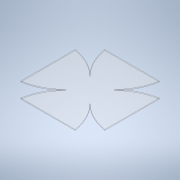
# Autodesk Inventor part: IMPRESION SIN PINES
Saved by Autodesk Inventor 2020 (Build 240168000, 168)
## iProperties
Created: 2021-11-17
Part Number: IMPRESION SIN PINES
Material: Plástico PET
Document SubType Name: Modeling
Designer: MATT
Density: 1.541 g/cm^3
Appearance: Policarbonato - Claro
Author: MATT
Autodesk Inventor part; units mm, degrees
ref_plane "YZ Plane" through (0, 0, 0) normal (1, 0, 0) x (0, 1, 0)
ref_plane "XZ Plane" through (0, 0, 0) normal (0, 1, 0) x (-1, 0, 0)
ref_plane "XY Plane" through (0, 0, 0) normal (0, 0, 1) x (1, 0, 0)
sketch "Boceto1" plane through (0, 0, 0) normal (0, 1, 0) x (-1, 0, 0)
  circle A0 centre (0, 0) radius 35
  line L0 (-85, 55) -> (-85, -55)
  line L1 (-55, -85) -> (55, -85)
  line L2 (85, -55) -> (85, 55)
  line L3 (55, 85) -> (-55, 85)
  arc A1 (24.7487, 24.7487) -> (55, 85) centre (-53.7007, 101.857) ccw
  arc A2 (85, 55) -> (24.7487, 24.7487) centre (101.857, -53.7007) ccw
  arc A3 (24.7487, -24.7487) -> (85, -55) centre (101.857, 53.7007) ccw
  arc A4 (55, -85) -> (24.7487, -24.7487) centre (-53.7007, -101.857) ccw
  arc A5 (-24.7487, -24.7487) -> (-55, -85) centre (53.7007, -101.857) ccw
  arc A6 (-85, -55) -> (-24.7487, -24.7487) centre (-101.857, 53.7007) ccw
  arc A7 (-24.7487, 24.7487) -> (-85, 55) centre (-101.857, -53.7007) ccw
  arc A8 (-55, 85) -> (-24.7487, 24.7487) centre (53.7007, 101.857) ccw
  dimension "d3" = 70
  constraints: 20 point on circle, 9 centre point, 8 end point, 1 horizontal, 1 perpendicular
  measures "d3" diameter of A0
extrude "Extrusión1" add sketch "Boceto1" along normal blind 2
